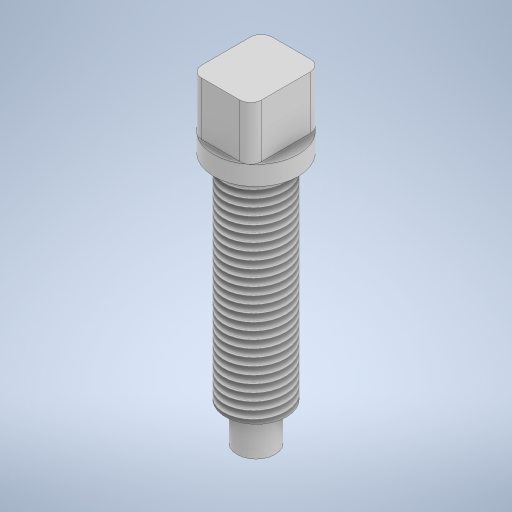
# Autodesk Inventor part: SetScrew
Saved by Autodesk Inventor 2024 (Build 280153000, 153)
## iProperties
Created: 2023-11-09
Part Number: SetScrew
Material: Generic
Document SubType Name: Modeling
Designer: Admin
Density: 1 g/cm^3
Appearance: Default
Author: Admin
Autodesk Inventor part; units mm, degrees
ref_plane "YZ Plane" through (0, 0, 0) normal (1, 0, 0) x (0, 1, 0)
ref_plane "XZ Plane" through (0, 0, 0) normal (0, 1, 0) x (-1, 0, 0)
ref_plane "XY Plane" through (0, 0, 0) normal (0, 0, 1) x (1, 0, 0)
sketch "Sketch1" plane through (0, 0, 0) normal (0, 1, 0) x (-1, 0, 0)
  circle A0 centre (0, 0) radius 8
  circle A1 centre (0, 0) radius 5
  dimension "d0" = 16
  dimension "d1" = 10
  constraints: 2 centre point, 2 coincident
  measures "d0" diameter of A0
  measures "d1" diameter of A1
extrude "Extrusion1" add sketch "Sketch1" along normal blind 56 contours A0 | A1
extrude "Extrusion2" add sketch "Sketch1" against normal blind 10 contours A1
sketch "Sketch2" plane through (0, 56, 0) normal (0, 1, 0) x (1, 0, 0)
  circle A0 centre (0, 0) radius 11
  dimension "d6" = 22
  constraints: 1 centre point, 1 coincident
  measures "d6" diameter of A0
extrude "Extrusion3" add sketch "Sketch2" along normal blind 5
sketch "Sketch3" plane through (0, 61, 0) normal (0, 1, 0) x (1, 0, 0)
  circle A0 centre (0, 0) radius 11 projected
  line L0 (-5.0525, -8.4417) -> (5.0525, -8.4417) construction
  line L1 (7.0525, -6.4417) -> (7.0525, 6.4417) construction
  line L2 (5.0525, 8.4417) -> (-5.0525, 8.4417) construction
  line L3 (-7.0525, 6.4417) -> (-7.0525, -6.4417) construction
  line L4 (-7.0525, -8.4417) -> (7.0525, 8.4417) construction
  line L5 (7.0525, -8.4417) -> (-7.0525, 8.4417) construction
  arc A1 (7.0525, 6.4417) -> (5.0525, 8.4417) centre (5.0525, 6.4417) ccw construction
  arc A2 (5.0525, -8.4417) -> (7.0525, -6.4417) centre (5.0525, -6.4417) ccw construction
  arc A3 (-7.0525, -6.4417) -> (-5.0525, -8.4417) centre (-5.0525, -6.4417) ccw construction
  arc A4 (-5.0525, 8.4417) -> (-7.0525, 6.4417) centre (-5.0525, 6.4417) ccw construction
  line L6 (7.8658, 6.4417) -> (7.8658, -6.4417)
  arc A5 (5.0525, -9.2549) -> (7.8658, -6.4417) centre (5.0525, -6.4417) ccw
  line L7 (5.0525, -9.2549) -> (-5.0525, -9.2549)
  arc A6 (-7.8658, -6.4417) -> (-5.0525, -9.2549) centre (-5.0525, -6.4417) ccw
  line L8 (-7.8658, -6.4417) -> (-7.8658, 6.4417)
  arc A7 (-5.0525, 9.2549) -> (-7.8658, 6.4417) centre (-5.0525, 6.4417) ccw
  line L9 (-5.0525, 9.2549) -> (5.0525, 9.2549)
  arc A8 (7.8658, 6.4417) -> (5.0525, 9.2549) centre (5.0525, 6.4417) ccw
  dimension "d9" = 2
  constraints: 20 end point, 17 point on circle, 9 tangent, 8 centre point, 8 point on line, 4 parallel, 3 equal radius, 2 midpoint, 2 perpendicular, 1 horizontal, 7 other
  measures "d9" radius of A1
extrude "Extrusion4" add sketch "Sketch3" along normal blind 14 contours A8 L6 A5 L7 A6 L8 A7 L9
thread "Thread1" size "M16x2" class "6g" standard "ANSI Metric M Profile" length 56
body "Solid1"
